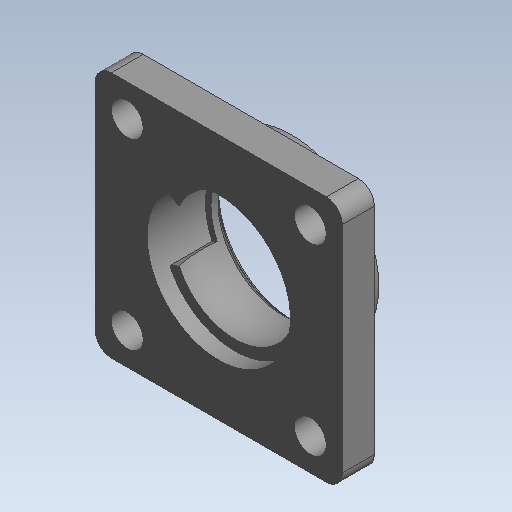
# Autodesk Inventor part: F4BSS 504-Y-housing
Saved by Autodesk Inventor 2020 (Build 240168000, 168)
## iProperties
Part Number: F4BSS 504-Y-housing
Material: Generic
Catalog Web Link: www.cadenas.de
Description: ayf_001hc_hh_hy-housing-Square flanged housings for Y-bearings
Vendor: SKF
Document SubType Name: Modeling
Designer: partserver
Manufacturer: SKF
Mass: 78.8047 g
Surface Area: 224.885 cm^2
Volume: 78.8047 cm^3
Density: 1 g/cm^3
Appearance: PSOLRGB-175-175-175
Category: PARTsolutions
Company: SKF
PSOL_IDENT_0: {$CADENAS_DATA\23d-libs\skf\bearings_units_and_housings\bearing_units\ball_bearing_units\y-units\y-b
PSOL_IDENT_1: earing_square_flanged_units_parts\ayf_001hc_hh_hy_housing.prj},202 {VTYP=3D},{NB=F4BSS 504-Y-housing
PSOL_IDENT_2: },{LINA=F4BSS 504-Y-housing},{NN=ayf_001hc_hh_hy-housing},{DATE=20.08.2020 13:45:19},{GEOMDATE=29.07
PSOL_IDENT_3: .2020 16:36:58},{VERSION=},{LINEID=9470},{WBVAR=COVER},{WBNUMERIC=}  {NB=F4BSS 504-Y-housing},{LINA=
PSOL_IDENT_4: F4BSS 504-Y-housing},{KT=DUMMY},{DESIGNATION=F4BSS 504-Y},{SS1=MIN},{T=MIN},{COVER=},{GN=},{D=47.000
PSOL_IDENT_5: },{DA=MIN},{DB1=MIN},{DB2=MIN},{DB=MIN},{A=25.800},{A1=11.100},{A2=MIN},{A3=MIN},{A5=25.400},{J=63.5
PSOL_IDENT_6: 00},{L=85.700},{N=11.100},{RG=},{R1=MIN},{DN=MIN},{SWN=MIN},{J6=MIN},{J7=MIN},{N4=MIN},{EC=ECW 204},
PSOL_IDENT_7: {AEC=29.000},{DEC=40.900},{D1EC=48.900},{D2EC=50.500},{E=14},{DESIGN=f4bss},{BRG=0.000},{ECPN=},{H4=
PSOL_IDENT_8: MIN},{R2=MIN},{R3=MIN},{R4=MIN},{L1=MIN},{H5=MIN},{R5=MIN},{H6=MIN},{L2=MIN},{H7=MIN},{H8=MIN},{H9=M
PSOL_IDENT_9: IN},{L3=MIN},{L4=MIN},{H10=MIN},{H11=MIN},{H12=MIN},{H13=MIN},{H14=MIN},{R6=MIN},{L5=MIN},{H15=MIN},
PSOL_IDENT_10: {H16=MIN},{SC=MIN}
NB: F4BSS 504-Y-housing
NN: ayf_001hc_hh_hy-housing
NT: Square flanged housings for Y-bearings
NBSYN: $DESIGNATION.$ECPN.-housing
LINA: F4BSS 504-Y-housing
CATALOG: SKF
DESIGNATION: F4BSS 504-Y
SS1: 0
T: 0
COVER: No End Cover
D: 47
DA: 0
DB1: 0
DB2: 0
DB: 0
A: 25.8
A1: 11.1
A2: 0
A3: 0
A5: 25.4
J: 63.5
L: 85.7
N: 11.1
R1: 0
DN: 0
SWN: 0
J6: 0
J7: 0
N4: 0
EC: ECW 204
AEC: 29
DEC: 40.9
D1EC: 48.9
D2EC: 50.5
DESIGN: f4bss
H4: 0
R2: 0
R3: 0
R4: 0
L1: 0
H5: 0
R5: 0
H6: 0
L2: 0
H7: 0
H8: 0
H9: 0
L3: 0
L4: 0
H10: 0
H11: 0
H12: 0
H13: 0
H14: 0
R6: 0
L5: 0
H15: 0
H16: 0
SC: 0
SUPPLIER: SKF
ARTICLENO: F4BSS 504-Y-housing
BOMINFO: F4BSS 504-Y-housing
CREATOR: CADENAS GmbH
Title: F4BSS 504-Y-housing
Author: Cadenas PARTsolutions
Comments: Square flanged housings for Y-bearings
Autodesk Inventor part; units mm, degrees
sketch "Sketch_1" plane through (0, 0, 0) normal (0, 0, 1) x (1, 0, 0)
  line L0 (0, 0) -> (0, 25.8)
  arc A0 (21.3361, 5.55) -> (21.0734, 25.8) centre (0, 15.4) ccw
  line L1 (21.3361, 5.55) -> (24.8875, 5.55)
  line L2 (24.8875, 5.55) -> (24.8875, 0)
  line L3 (24.8875, 0) -> (85.7, 0)
  line L4 (85.7, 0) -> (85.7, 9.1)
  arc A1 (85.7, 9.1) -> (83.7, 11.1) centre (83.7, 9.1) ccw
  line L5 (83.7, 11.1) -> (33.4994, 11.1)
  arc A2 (33.4994, 11.1) -> (30.2815, 25.2277) centre (0, 10.9) ccw
  arc A3 (30.2815, 25.2277) -> (29.3775, 25.8) centre (29.3775, 24.8) ccw
  line L6 (29.3775, 25.8) -> (21.0734, 25.8)
  constraints: 14 end point, 8 point on circle, 4 centre point
revolve "Revolution1" add sketch "Sketch_1" angle 360 about axis through (0, 0, 0) along (0, -1, 0)
sketch "Sketch_6" plane through (0, 0, 0) normal (0, 1, 0) x (-1, 0, 0)
  circle A0 centre (0, 0) radius 87.7
  arc A1 (42.85, 37.3) -> (37.3, 42.85) centre (37.3, 37.3) ccw
  line L0 (37.3, 42.85) -> (-37.3, 42.85)
  arc A2 (-37.3, 42.85) -> (-42.85, 37.3) centre (-37.3, 37.3) ccw
  line L1 (-42.85, 37.3) -> (-42.85, -37.3)
  arc A3 (-42.85, -37.3) -> (-37.3, -42.85) centre (-37.3, -37.3) ccw
  line L2 (-37.3, -42.85) -> (37.3, -42.85)
  arc A4 (37.3, -42.85) -> (42.85, -37.3) centre (37.3, -37.3) ccw
  line L3 (42.85, -37.3) -> (42.85, 37.3)
  constraints: 8 end point, 8 point on circle, 5 centre point
extrude "Extrusion1" cut sketch "Sketch_6" along normal blind 25.8
sketch "Sketch_7" plane through (0, 0, 42.85) normal (0, 0, 1) x (1, 0, 0)
  arc A0 (-5.55, 10.2565) -> (5.55, 10.2565) centre (0, 16.32) ccw
  line L0 (5.55, 10.2565) -> (5.55, 11.1)
  line L1 (5.55, 11.1) -> (-5.55, 11.1)
  line L2 (-5.55, 11.1) -> (-5.55, 10.2565)
  constraints: 6 end point, 2 point on circle, 1 centre point
extrude "Extrusion2" cut sketch "Sketch_7" against normal blind 12.85
sketch "Sketch_4" plane through (0, 0, 0) normal (0, 0, 1) x (1, 0, 0)
  line L0 (0, 5.55) -> (0, 20.25)
  line L1 (0, 20.25) -> (24.8875, 20.25)
  line L2 (24.8875, 20.25) -> (24.8875, 5.55)
  line L3 (24.8875, 5.55) -> (0, 5.55)
  line L4 (0, 5.55) -> (0, 20.25)
  constraints: 10 end point
revolve "Revolution2" cut sketch "Sketch_4" angle 50 mid plane about axis through (0, 5.55, 0) along (0, 1, 0)
sketch "Sketch_5" plane through (0, 0, 0) normal (0, 0, 1) x (1, 0, 0)
  line L0 (0, 14.7) -> (0, -5.55)
  line L1 (0, -5.55) -> (-24.8875, -5.55)
  line L2 (-24.8875, -5.55) -> (-24.8875, 14.7)
  line L3 (-24.8875, 14.7) -> (0, 14.7)
  line L4 (0, 14.7) -> (0, -5.55)
  constraints: 10 end point
revolve "Revolution3" cut sketch "Sketch_5" angle 50 mid plane about axis through (0, 14.7, 0) along (0, -1, 0)
sketch "Sketch6" plane through (-37.3, 11.1, -42.85) normal (0, 1, 0) x (1, 0, 0)
  point P0 (5.55, -11.1)
hole "Hole1" at (-31.75, 11.1, -31.75) direction (0, -1, 0) diameter 11.1 depth 11.1
pattern_linear "Rectangular Pattern1" count 2 spacing 63.5 along (1, 0, 0) count 2 spacing 63.5 along (0, 0, 1) of "Hole1"
sketch "Sketch_9" plane through (0, 0, 0) normal (0, 0, 1) x (1, 0, 0)
  line L0 (0, 25.8) -> (0, 22.2)
  line L1 (0, 22.2) -> (-24.25, 22.2)
  arc A0 (-25.2242, 23.4257) -> (-24.25, 22.2) centre (-24.25, 23.2) ccw
  arc A1 (-24.9537, 23.834) -> (-25.2242, 23.4257) centre (-24.5423, 23.2677) ccw
  line L2 (-24.9537, 23.834) -> (-24.45, 24.2)
  line L3 (-24.45, 24.2) -> (-24.4698, 24.361)
  line L4 (-24.4698, 24.361) -> (-25.9088, 25.8)
  line L5 (-25.9088, 25.8) -> (0, 25.8)
  line L6 (0, 25.8) -> (0, 22.2)
  constraints: 14 end point, 4 point on circle, 2 centre point
revolve "Revolution4" cut sketch "Sketch_9" angle 360 about axis through (0, 25.8, 0) along (0, 1, 0)
sketch "Sketch_10" plane through (0, 0, 33.5) normal (0, 0, 1) x (1, 0, 0)
  line L0 (-5.55, 25.8) -> (-5.55, 6.1)
  line L1 (-5.55, 6.1) -> (5.55, 6.1)
  line L2 (5.55, 6.1) -> (5.55, 25.8)
  line L3 (5.55, 25.8) -> (-5.55, 25.8)
  constraints: 8 end point
extrude "Extrusion3" add sketch "Sketch_10" against normal blind 5.55
ref_plane "brg_XY" through (0, 12.9, 0) normal (0, 1, 0) x (1, 0, 0)
ref_plane "brg_YZ" through (0, 12.9, 0) normal (1, 0, 0) x (0, 0, -1)
ref_plane "brg_ZX" through (0, 12.9, 0) normal (0, 0, -1) x (0, 1, 0)
ref_plane "housing_XY" through (0, 0, 0) normal (0, 1, 0) x (1, 0, 0)
ref_plane "housing_YZ" through (0, 0, 0) normal (1, 0, 0) x (0, 0, -1)
ref_plane "housing_ZX" through (0, 0, 0) normal (0, 0, -1) x (0, 1, 0)
ref_plane "tocover_XY" through (0, 51.2, 0) normal (0, 1, 0) x (1, 0, 0)
ref_plane "tocover_YZ" through (0, 51.2, 0) normal (1, 0, 0) x (0, 0, -1)
ref_plane "tocover_ZX" through (0, 51.2, 0) normal (0, 0, -1) x (0, 1, 0)
body "Solid1"
